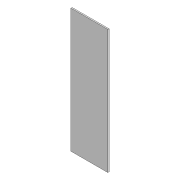
# Autodesk Inventor part: Back
Saved by Autodesk Inventor 2021.3 (Build 253353000, 353)
## iProperties
Created: 2021-11-26
Part Number: Back
Material: Generic
Document SubType Name: Modeling
Designer: wbrooks
Density: 1 g/cm^3
Appearance: Default
Author: wbrooks
Autodesk Inventor part; units mm, degrees
ref_plane "YZ Plane" through (0, 0, 0) normal (1, 0, 0) x (0, 1, 0)
ref_plane "XZ Plane" through (0, 0, 0) normal (0, 1, 0) x (-1, 0, 0)
ref_plane "XY Plane" through (0, 0, 0) normal (0, 0, 1) x (1, 0, 0)
sketch "Sketch1" plane through (0, 0, 0) normal (0, 0, 1) x (1, 0, 0)
  line L0 (180.975, 609.6) -> (-180.975, 609.6)
  line L1 (-180.975, 609.6) -> (-180.975, -609.6)
  line L2 (-180.975, -609.6) -> (180.975, -609.6)
  line L3 (180.975, -609.6) -> (180.975, 609.6)
  line L4 (180.975, 609.6) -> (-180.975, -609.6) construction
  line L5 (-180.975, 609.6) -> (180.975, -609.6) construction
  point P0 (0, 0)
  dimension "d2" = 361.95
  dimension "d3" = 1219.2
  constraints: 12 end point, 2 midpoint, 2 parallel, 1 horizontal, 1 perpendicular
  measures "d2" distance of L0.start L0.end
  measures "d3" distance of L2.end L0.start
extrude "Extrusion1" add sketch "Sketch1" along normal mid plane 11.9062
body "Solid1"
